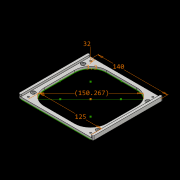
# Autodesk Inventor part: bottom_140mm_2
Saved by Autodesk Inventor 2018 (Build 220112000, 112)
## iProperties
Created: 2022-10-02
Part Number: bottom_140mm_2
Material: アルミニウム 6061
Document SubType Name: Modeling
Designer: gisen
Density: 2.7 g/cm^3
Appearance: アルミニウム - フラット
Author: gisen
Autodesk Inventor part; units mm, degrees
ref_plane "YZ Plane" through (0, 0, 0) normal (1, 0, 0) x (0, 1, 0)
ref_plane "XZ Plane" through (0, 0, 0) normal (0, 1, 0) x (-1, 0, 0)
ref_plane "XY Plane" through (0, 0, 0) normal (0, 0, 1) x (1, 0, 0)
sketch "スケッチ1" plane through (0, 0, 0) normal (0, 0, 1) x (1, 0, 0)
  line L0 (-70, 70) -> (70, 70)
  line L1 (70, 70) -> (70, -70)
  line L2 (70, -70) -> (-70, -70)
  line L3 (-70, -70) -> (-70, 70)
  line L4 (-62.5, 62.5) -> (62.5, 62.5) construction
  line L5 (62.5, 62.5) -> (62.5, -62.5) construction
  line L6 (62.5, -62.5) -> (-62.5, -62.5) construction
  line L7 (-62.5, -62.5) -> (-62.5, 62.5) construction
  circle A0 centre (-62.5, 62.5) radius 1.65
  line L8 (-30.5, 62.5) -> (30.5, 62.5)
  line L9 (62.5, 30.5) -> (62.5, -30.5)
  line L10 (30.5, -62.5) -> (-30.5, -62.5)
  line L11 (-62.5, -30.5) -> (-62.5, 30.5)
  arc A1 (-30.5, 62.5) -> (-62.5, 30.5) centre (-30.5, 30.5) ccw
  arc A2 (-62.5, -30.5) -> (-30.5, -62.5) centre (-30.5, -30.5) ccw
  arc A3 (30.5, -62.5) -> (62.5, -30.5) centre (30.5, -30.5) ccw
  arc A4 (62.5, 30.5) -> (30.5, 62.5) centre (30.5, 30.5) ccw
  line L12 (53.1274, 53.1274) -> (-53.1274, -53.1274) construction
  circle A5 centre (-62.5, -62.5) radius 1.65
  circle A6 centre (62.5, -62.5) radius 1.65
  circle A7 centre (62.5, 62.5) radius 1.65
  point P0 (0, 0)
  point P1 (-70, 0)
  point P2 (0, 70)
  point P3 (-62.5, 0)
  point P4 (0, 62.5)
  dimension "d0" = 140
  dimension "d1" = 125
  dimension "d3" = 3.3
  dimension "d4" = 32
  dimension "d5" = 150.267
  constraints: 26 end point, 10 point on circle, 8 centre point, 8 tangent, 6 equal radius, 6 midpoint, 6 parallel, 5 perpendicular, 4 coincident, 3 horizontal, 2 horizontal alignment, 2 point on line, 2 vertical alignment
  measures "d0" distance of L0.start L0.end
  measures "d1" distance of L5.end L6.end
  measures "d3" diameter of A0
  measures "d4" radius of A1
  measures "d5" distance of L12.start L12.end
extrude "押し出し1" add sketch "スケッチ1" along normal blind 4
sketch "スケッチ2" plane through (0, 0, 4) normal (0, 0, 1) x (1, 0, 0)
  line L0 (-70, 70) -> (-70, -70) construction
  line L1 (70, -70) -> (70, 70) construction
  line L2 (-70, 70) -> (-75, 70)
  line L3 (-75, 70) -> (-75, -70)
  line L4 (-75, -70) -> (-70, -70)
  line L5 (-70, -70) -> (-70, 70)
  line L6 (70, 70) -> (75, 70)
  line L7 (75, 70) -> (75, -70)
  line L8 (75, -70) -> (70, -70)
  line L9 (70, -70) -> (70, 70)
  point P0 (0, 0)
  dimension "d8" = 150
  constraints: 16 end point, 4 parallel, 2 equal length, 2 horizontal, 2 perpendicular
  measures "d8" distance between parallel lines of L7 L3
extrude "押し出し2" add sketch "スケッチ2" against normal up to surface (4 mm away)
sketch "スケッチ3" plane through (0, 0, 4) normal (0, 0, 1) x (1, 0, 0)
  line L0 (-75, 70) -> (-75, -70) construction
  line L1 (75, 70) -> (75, -70) construction
  line L2 (-75, 70) -> (-70.2, 70)
  line L3 (-70.2, 70) -> (-70.2, -70)
  line L4 (-70.2, -70) -> (-75, -70)
  line L5 (-75, -70) -> (-75, 70)
  line L6 (75, 70) -> (70.2, 70)
  line L7 (70.2, 70) -> (70.2, -70)
  line L8 (70.2, -70) -> (75, -70)
  line L9 (75, -70) -> (75, 70)
  point P0 (0, 0)
  dimension "d11" = 140.4
  constraints: 16 end point, 4 parallel, 2 horizontal, 2 perpendicular, 1 collinear
  measures "d11" distance between parallel lines of L7 L3
extrude "押し出し3" add sketch "スケッチ3" along normal blind 4
sketch "スケッチ5" plane through (0, 0, 0) normal (0, 0, -1) x (-1, 0, 0)
  line L0 (75, -70) -> (75, 70) construction
  line L1 (-75, 70) -> (-75, -70) construction
  line L2 (65, -70) -> (65, 70) construction
  line L3 (-65, 70) -> (-65, -70) construction
  circle A0 centre (65, -50) radius 2.25
  circle A1 centre (-65, -50) radius 2.25
  circle A2 centre (65, 50) radius 2.25
  circle A3 centre (-65, 50) radius 2.25
  circle A4 centre (65, -50) radius 7.5 construction
  point P0 (0, 0)
  dimension "d14" = 10
  dimension "d15" = 10
  dimension "d16" = 4.5
  dimension "d17" = 50
  dimension "d18" = 50
  dimension "d19" = 15
  constraints: 5 centre point, 4 end point, 4 point on line, 3 equal radius, 2 horizontal alignment, 2 parallel, 1 coincident
  measures "d14" distance between parallel lines of L0 L2
  measures "d15" distance between parallel lines of L1 L3
  measures "d16" diameter of A0
  measures "d17" vertical distance of point (0, 0) A0.centre
  measures "d18" vertical distance of A2.centre point (0, 0)
  measures "d19" diameter of A4
extrude "押し出し4" cut sketch "スケッチ5" against normal through all
sketch "スケッチ6" plane through (0, 0, 4) normal (0, 0, 1) x (1, 0, 0)
  circle A0 centre (-65, -50) radius 2.25 construction
  circle A1 centre (65, -50) radius 2.25 construction
  circle A2 centre (65, 50) radius 2.25 construction
  circle A3 centre (-65, 50) radius 2.25 construction
  circle A4 centre (-65, -50) radius 4.25
  circle A5 centre (-65, 50) radius 4.25
  circle A6 centre (65, -50) radius 4.25
  circle A7 centre (65, 50) radius 4.25
  point P0 (0, 0)
  dimension "d22" = 8.5
  constraints: 4 centre point, 4 coincident, 3 equal radius
  measures "d22" diameter of A4
extrude "押し出し5" cut sketch "スケッチ6" against normal blind 1.5
fillet "フィレット1" radius 2 8 edges at (75, 70, 4) (70.2, 70, 6) (75, -70, 4) (70.2, -70, 6) (-70.2, -70, 6) (-75, -70, 4) (-75, 70, 4) (-70.2, 70, 6)
equation "\"d18\" = d17"
